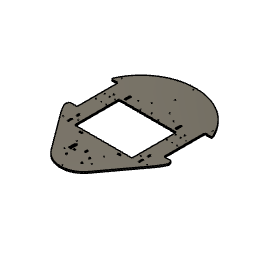
move_base_main_plate (Autodesk Fusion 360 design; units mm, degrees)
Autodesk Fusion 360 part; units mm, degrees
note: some values were not read from the file. Set by a fixed rule: which sketch regions a step uses.
sketch "スケッチ1" plane through (0, 0, 0) normal (0, 1, 0) x (1, 0, 0)
  circle A0 centre (0, 0) radius 210
  circle A1 centre (0, -210) radius 85
  line L0 (-168.7454, -125) -> (-68.3017, -260.5952)
  line L1 (68.3017, -260.5952) -> (168.7454, -125)
  circle A2 centre (0, 0) radius 200
  dimension "d1" = 420
  dimension "d2" = 210
  dimension "d3" = 170
  dimension "d4" = 400
  constraint coincident A0.centre A2.centre
  constraint vertical A0.centre A1.centre
  constraint tangent A0 L1
  constraint tangent A1 L1
  constraint tangent A1 L0
  constraint tangent A0 L0
  constraint coincident A0 L0.start
  constraint coincident A1 L0.end
  constraint coincident A1 L1.start
  constraint coincident A0 L1.end
  measures "d1" diameter of A0
  measures "d2" distance of A0.centre A1.centre
  measures "d3" diameter of A1
  measures "d4" diameter of A2
sketch "スケッチ2" plane through (0, 0, 0) normal (0, 1, 0) x (1, 0, 0)
  arc A0 (185.405, 75) -> (-185.405, 75) centre (0, 0) ccw
  arc A1 (-68.3017, -260.5952) -> (68.3017, -260.5952) centre (0, -210) ccw
  circle A2 centre (0, 0) radius 200
  line L0 (-185.405, 75) -> (-159, 75)
  line L1 (-159, 75) -> (-159, -75)
  line L2 (185.405, 75) -> (159, 75)
  line L3 (159, 75) -> (159, -75)
  line L4 (159, -75) -> (196.1505, -75)
  arc A3 (-196.1505, -75) -> (-168.7454, -125) centre (0, 0) ccw
  arc A4 (168.7454, -125) -> (196.1505, -75) centre (0, 0) ccw
  circle A5 centre (0, 0) radius 210
  line L5 (-168.7454, -125) -> (-68.3017, -260.5952)
  line L6 (68.3017, -260.5952) -> (168.7454, -125)
  line L7 (-196.1505, -75) -> (-159, -75)
  point P0 (-168.7454, -125)
  point P1 (-68.3017, -260.5952)
  point P2 (68.3017, -260.5952)
  point P3 (168.7454, -125)
  point P4 (0, -210)
  point P5 (-159, 0)
  point P6 (159, 0)
  dimension "d5" = 159
  dimension "d6" = 159
  dimension "d7" = 150
  dimension "d8" = 150
  constraint coincident A0.centre A2.centre
  constraint coincident A0.start A2
  constraint horizontal L0
  constraint perpendicular L0 L1
  constraint horizontal L2
  constraint perpendicular L2 L3
  constraint perpendicular L3 L4
  constraint coincident A3.start A5
  constraint coincident L4.end A5
  constraint coincident P0 A3.end
  constraint coincident P1 A1.start
  constraint coincident P2 A1.end
  constraint coincident P3 A4.start
  constraint horizontal L7
  constraint coincident L1.end L7.end
  constraint coincident L4.end A4.end
  constraint coincident A1.centre P4
  constraint midpoint L1 P5
  constraint midpoint L3 P6
  constraint horizontal P5 A0.centre
  constraint horizontal P6 A0.centre
  measures "d5" distance of L1 A0.centre
  measures "d6" distance of L3 A0.centre
  measures "d7" distance of L0.end L1.end
  measures "d8" distance of L2.end L3.end
extrude "押し出し1" add sketch "スケッチ2" along normal blind 5 contours A0 A2 L0 L1 L2 L3 L4 L7 | A2 L4 A3 A4 A5 L7 | A1 A5 L5 L6
sketch "スケッチ3" plane through (0, 5, 0) normal (0, 1, 0) x (-1, 0, 0)
  arc A0 (-185.405, -75) -> (185.405, -75) centre (0, 0) ccw
  line L0 (185.405, -75) -> (159, -75)
  line L1 (159, -75) -> (159, 75)
  line L2 (159, 75) -> (196.1505, 75)
  arc A1 (196.1505, 75) -> (168.7454, 125) centre (0, 0) ccw
  line L3 (168.7454, 125) -> (68.3017, 260.5952)
  arc A2 (68.3017, 260.5952) -> (-68.3017, 260.5952) centre (0, 210) ccw
  line L4 (-68.3017, 260.5952) -> (-168.7454, 125)
  arc A3 (-168.7454, 125) -> (-196.1505, 75) centre (0, 0) ccw
  line L5 (-196.1505, 75) -> (-159, 75)
  line L6 (-159, 75) -> (-159, -75)
  line L7 (-159, -75) -> (-185.405, -75)
  line L8 (-130, -70) -> (130, -70)
  line L9 (130, -70) -> (130, 150)
  line L10 (130, 150) -> (-130, 150)
  line L11 (-130, 150) -> (-130, -70)
  line L12 (-130, -70) -> (130, 150) construction
  line L13 (130, -70) -> (-130, 150) construction
  line L14 (149.05, -15.6) -> (110.95, -15.6)
  line L15 (110.95, -15.6) -> (110.95, 15.6)
  line L16 (110.95, 15.6) -> (149.05, 15.6)
  line L17 (149.05, 15.6) -> (149.05, -15.6)
  line L18 (-110.95, -15.6) -> (-149.05, -15.6)
  line L19 (-149.05, -15.6) -> (-149.05, 15.6)
  line L20 (-149.05, 15.6) -> (-110.95, 15.6)
  line L21 (-110.95, 15.6) -> (-110.95, -15.6)
  line L22 (0, 200) -> (0, 260)
  arc A4 (-166.2769, -96) -> (166.2769, -96) centre (0, 0) ccw
  line L23 (0, 0) -> (0, -192)
  line L24 (0, 0) -> (-166.2769, -96)
  line L25 (0, 0) -> (166.2769, -96)
  line L26 (0, 260) -> (0, 287)
  line L27 (154.1352, 131.2832) -> (61.8733, 255.8333)
  arc A5 (61.8733, 255.8333) -> (-61.8733, 255.8333) centre (0, 210) ccw
  line L28 (-154.1352, 131.2832) -> (-61.8733, 255.8333)
  line L29 (0, 210) -> (61.8733, 255.8333)
  line L30 (0, 210) -> (-61.8733, 255.8333)
  line L31 (-28, 216) -> (28, 216)
  line L32 (28, 216) -> (28, 244)
  line L33 (28, 244) -> (-28, 244)
  line L34 (-28, 244) -> (-28, 216)
  line L35 (-28, 216) -> (28, 244) construction
  line L36 (28, 216) -> (-28, 244) construction
  line L37 (114.5, 115) -> (114.5, -54.5)
  line L38 (114.5, -54.5) -> (-114.5, -54.5)
  line L39 (-114.5, -54.5) -> (-114.5, 115)
  line L40 (33, -73) -> (-33, -73)
  line L41 (-33, -73) -> (-33, -31.5)
  line L42 (-33, -31.5) -> (33, -31.5)
  line L43 (33, -31.5) -> (33, -73)
  line L44 (128, 122) -> (132, 122)
  line L45 (132, 122) -> (132, 138)
  line L46 (132, 138) -> (128, 138)
  line L47 (128, 138) -> (128, 122)
  line L48 (128, 122) -> (132, 138) construction
  line L49 (132, 122) -> (128, 138) construction
  line L50 (-132, 122) -> (-128, 122)
  line L51 (-128, 122) -> (-128, 138)
  line L52 (-128, 138) -> (-132, 138)
  line L53 (-132, 138) -> (-132, 122)
  line L54 (-132, 122) -> (-128, 138) construction
  line L55 (-128, 122) -> (-132, 138) construction
  point P0 (0, 40)
  point P1 (130, -15.6)
  point P2 (-130, -15.6)
  point P3 (110.95, 0)
  point P4 (-110.95, 0)
  point P5 (70, -70)
  point P6 (-70, -70)
  point P7 (130, -30)
  point P8 (130, 100)
  point P9 (70, 150)
  point P10 (-70, 150)
  point P11 (-130, 100)
  point P12 (-130, -30)
  point P13 (0, 230)
  point P14 (130, 15.6)
  point P15 (-130, 15.6)
  point P16 (65, -54.5)
  point P17 (-65, -54.5)
  point P18 (0, -40)
  point P19 (0, -73)
  point P20 (0, 256)
  point P21 (0, -125)
  point P22 (130, 130)
  point P23 (-130, 130)
  dimension "d13" = 260
  dimension "d14" = 220
  dimension "d15" = 40
  dimension "d16" = 70
  dimension "d17" = 60
  dimension "d18" = 70
  dimension "d19" = 70
  dimension "d20" = 50
  dimension "d21" = 60
  dimension "d22" = 38.1
  dimension "d23" = 31.2
  dimension "d24" = 192
  dimension "d25" = 60
  dimension "d26" = 60
  dimension "d28" = 27
  dimension "d29" = 77
  dimension "d30" = 155
  dimension "d31" = 155
  dimension "d32" = 53.5
  dimension "d33" = 230
  dimension "d34" = 28
  dimension "d35" = 56
  dimension "d56" = 15.5
  dimension "d57" = 15.5
  dimension "d58" = 15.5
  dimension "d59" = 115
  dimension "d60" = 65
  dimension "d61" = 65
  dimension "d65" = 66
  dimension "d66" = 41.5
  dimension "d99" = 85
  dimension "d100" = 40
  dimension "d116" = 4
  dimension "d117" = 16
  dimension "d134" = 3
  dimension "d145" = 130
  constraint horizontal L8
  constraint perpendicular L8 L9
  constraint parallel L8 L10
  constraint parallel L9 L11
  constraint coincident L12 P0
  constraint coincident L13 P0
  constraint vertical A0.centre P0
  constraint horizontal L14
  constraint vertical L15
  constraint horizontal L16
  constraint vertical L17
  constraint midpoint L14 P1
  constraint coincident L9 P1
  constraint horizontal L18
  constraint vertical L19
  constraint horizontal L20
  constraint vertical L21
  constraint midpoint L18 P2
  constraint coincident L11 P2
  constraint midpoint L21 P4
  constraint midpoint L15 P3
  constraint horizontal A0.centre P3
  constraint horizontal A0.centre P4
  constraint coincident L8 P5
  constraint coincident L8 P6
  constraint coincident L9 P8
  constraint coincident L10 P9
  constraint coincident L10 P10
  constraint coincident L11 P11
  constraint coincident L11 P12
  constraint vertical P5 P9
  constraint vertical P6 P10
  constraint horizontal P7 P12
  constraint horizontal P8 P11
  constraint parallel L9 L22
  constraint vertical A0.centre L22.start
  constraint equal L14 L18
  constraint equal L15 L19
  constraint coincident A0.centre A1.centre
  constraint coincident A4 L23.end
  constraint vertical L23
  constraint parallel L22 L26
  constraint coincident A2.centre A5.centre
  constraint coincident L27.end A5.start
  constraint coincident A5.end L28.end
  constraint tangent L27 A5
  constraint tangent A5 L28
  constraint parallel L4 L28
  constraint parallel L3 L27
  constraint horizontal L31
  constraint perpendicular L31 L32
  constraint parallel L31 L33
  constraint parallel L32 L34
  constraint coincident L35 P13
  constraint coincident L36 P13
  constraint vertical A0.centre P13
  constraint midpoint L16 P14
  constraint midpoint L20 P15
  constraint vertical L37
  constraint perpendicular L23 L38
  constraint perpendicular L38 L39
  constraint coincident L38 P16
  constraint coincident L38 P17
  constraint vertical A0.centre P18
  constraint horizontal L40
  constraint vertical L41
  constraint horizontal L42
  constraint vertical L43
  constraint coincident L40 P19
  constraint midpoint L40 P19
  constraint vertical A0.centre P19
  constraint coincident L26 P20
  constraint coincident L23 P21
  constraint horizontal L44
  constraint perpendicular L44 L45
  constraint parallel L44 L46
  constraint parallel L45 L47
  constraint coincident L48 P22
  constraint coincident L49 P22
  constraint coincident L9 P22
  constraint horizontal L50
  constraint perpendicular L50 L51
  constraint parallel L50 L52
  constraint parallel L51 L53
  constraint coincident L54 P23
  constraint coincident L55 P23
  constraint coincident L11 P23
  constraint equal L44 L50
  constraint equal L47 L51
  constraint horizontal L37.start L39.end
  constraint horizontal P22 P23
  measures "d13" distance of L8.start L8.end
  measures "d14" distance of L8.start L10.end
  measures "d15" distance of A0.centre P0
  measures "d16" vertical distance of P0 P7
  measures "d17" vertical distance of P0 P8
  measures "d18" horizontal distance of P0 P9
  measures "d19" horizontal distance of P0 P10
  measures "d20" distance of L10 L22.start
  measures "d21" distance of L22.start L22.end
  measures "d22" distance of L14.start L14.end
  measures "d23" distance of L14.end L15.end
  measures "d24" radius of A4
  measures "d25" angle of L23 L24
  measures "d26" angle of L23 L25
  measures "d28" distance of L22.end L26.end
  measures "d29" radius of A5
  measures "d30" distance of L28.start A5.end
  measures "d31" distance of L27.start L27.end
  measures "d33" distance of A0.centre P13
  measures "d34" distance of L31.start L33.end
  measures "d35" distance of L32.end L33.end
  measures "d56" distance of L9 L37
  measures "d57" distance of L11 L39
  measures "d58" distance of L8 L38
  measures "d59" vertical distance of A0.centre L37.start
  measures "d60" horizontal distance of A0.centre P16
  measures "d61" horizontal distance of A0.centre P17
  measures "d65" distance of L40.start L40.end
  measures "d66" distance of L40.start L42.end
  measures "d99" distance of P18 P21
  measures "d100" distance of A0.centre P18
  measures "d116" distance of L44.start L44.end
  measures "d117" distance of L44.end L45.end
  measures "d134" distance of L8 L40
  measures "d145" vertical distance of A0.centre P22
hole "穴1" at (-166.2769, 5, -96) at (0, 5, -192) at (166.2769, 5, -96) at (149.05, 5, -15.6) at (149.05, 5, 15.6) at (110.95, 5, -15.6) at (110.95, 5, 15.6) at (-110.95, 5, -15.6) at (-149.05, 5, -15.6) at (-149.05, 5, 15.6) at (-110.95, 5, 15.6) at (-130, 5, -15.6) at (130, 5, -15.6) at (130, 5, 15.6) at (-130, 5, 15.6) at (-154.1352, 5, 131.2832) at (0, 5, 287) at (154.1352, 5, 131.2832) at (-114.5, 5, 115) at (-65, 5, -54.5) at (65, 5, -54.5) at (114.5, 5, 115) at (-33, 5, -31.5) at (33, 5, -31.5) at (33, 5, -73) at (-33, 5, -73) at (0, 5, -40) at (0, 5, -125) direction (0, -1, 0) diameter 3.2 end through all
sketch "スケッチ4" plane through (0, 5, 0) normal (0, 1, 0) x (-1, 0, 0)
  circle A0 centre (0, 287) radius 1.6
  circle A1 centre (130, 15.6) radius 1.6
  circle A2 centre (-130, -15.6) radius 1.6
  circle A3 centre (110.95, 15.6) radius 1.6
  circle A4 centre (149.05, -15.6) radius 1.6
  circle A5 centre (-110.95, 15.6) radius 1.6
  circle A6 centre (-149.05, 15.6) radius 1.6
  circle A7 centre (-166.2769, -96) radius 1.6
  circle A8 centre (166.2769, -96) radius 1.6
  circle A9 centre (0, -192) radius 1.6
  circle A10 centre (-149.05, -15.6) radius 1.6
  circle A11 centre (-110.95, -15.6) radius 1.6
  circle A12 centre (110.95, -15.6) radius 1.6
  circle A13 centre (149.05, 15.6) radius 1.6
  circle A14 centre (130, -15.6) radius 1.6
  circle A15 centre (-130, 15.6) radius 1.6
  circle A16 centre (154.1352, 131.2832) radius 1.6
  circle A17 centre (-154.1352, 131.2832) radius 1.6
  arc A18 (-185.405, -75) -> (185.405, -75) centre (0, 0) ccw
  line L0 (185.405, -75) -> (159, -75)
  line L1 (159, -75) -> (159, 75)
  line L2 (159, 75) -> (196.1505, 75)
  arc A19 (196.1505, 75) -> (168.7454, 125) centre (0, 0) ccw
  line L3 (168.7454, 125) -> (68.3017, 260.5952)
  arc A20 (68.3017, 260.5952) -> (-68.3017, 260.5952) centre (0, 210) ccw
  line L4 (-68.3017, 260.5952) -> (-168.7454, 125)
  arc A21 (-168.7454, 125) -> (-196.1505, 75) centre (0, 0) ccw
  line L5 (-196.1505, 75) -> (-159, 75)
  line L6 (-159, 75) -> (-159, -75)
  line L7 (-159, -75) -> (-185.405, -75)
  line L8 (127.85, -34) -> (132.15, -34)
  line L9 (132.15, -34) -> (132.15, -26)
  line L10 (132.15, -26) -> (127.85, -26)
  line L11 (127.85, -26) -> (127.85, -34)
  line L12 (127.85, -34) -> (132.15, -26) construction
  line L13 (132.15, -34) -> (127.85, -26) construction
  circle A22 centre (130, -34) radius 2.15
  circle A23 centre (130, -26) radius 2.15
  line L14 (127.85, 96) -> (132.15, 96)
  line L15 (132.15, 96) -> (132.15, 104)
  line L16 (132.15, 104) -> (127.85, 104)
  line L17 (127.85, 104) -> (127.85, 96)
  line L18 (127.85, 96) -> (132.15, 104) construction
  line L19 (132.15, 96) -> (127.85, 104) construction
  line L20 (-132.15, 96) -> (-127.85, 96)
  line L21 (-127.85, 96) -> (-127.85, 104)
  line L22 (-127.85, 104) -> (-132.15, 104)
  line L23 (-132.15, 104) -> (-132.15, 96)
  line L24 (-132.15, 96) -> (-127.85, 104) construction
  line L25 (-127.85, 96) -> (-132.15, 104) construction
  line L26 (-132.15, -34) -> (-127.85, -34)
  line L27 (-127.85, -34) -> (-127.85, -26)
  line L28 (-127.85, -26) -> (-132.15, -26)
  line L29 (-132.15, -26) -> (-132.15, -34)
  line L30 (-132.15, -34) -> (-127.85, -26) construction
  line L31 (-127.85, -34) -> (-132.15, -26) construction
  line L32 (66, 147.85) -> (74, 147.85)
  line L33 (74, 147.85) -> (74, 152.15)
  line L34 (74, 152.15) -> (66, 152.15)
  line L35 (66, 152.15) -> (66, 147.85)
  line L36 (66, 147.85) -> (74, 152.15) construction
  line L37 (74, 147.85) -> (66, 152.15) construction
  line L38 (-74, 147.85) -> (-66, 147.85)
  line L39 (-66, 147.85) -> (-66, 152.15)
  line L40 (-66, 152.15) -> (-74, 152.15)
  line L41 (-74, 152.15) -> (-74, 147.85)
  line L42 (-74, 147.85) -> (-66, 152.15) construction
  line L43 (-66, 147.85) -> (-74, 152.15) construction
  circle A24 centre (-130, -34) radius 2.15
  circle A25 centre (-130, -26) radius 2.15
  circle A26 centre (-130, 96) radius 2.15
  circle A27 centre (-130, 104) radius 2.15
  circle A28 centre (-74, 150) radius 2.15
  circle A29 centre (-66, 150) radius 2.15
  circle A30 centre (66, 150) radius 2.15
  circle A31 centre (74, 150) radius 2.15
  circle A32 centre (130, 96) radius 2.15
  circle A33 centre (130, 104) radius 2.15
  line L44 (-2.15, 196) -> (2.15, 196)
  line L45 (2.15, 196) -> (2.15, 204)
  line L46 (2.15, 204) -> (-2.15, 204)
  line L47 (-2.15, 204) -> (-2.15, 196)
  line L48 (-2.15, 196) -> (2.15, 204) construction
  line L49 (2.15, 196) -> (-2.15, 204) construction
  circle A34 centre (0, 196) radius 2.15
  circle A35 centre (0, 204) radius 2.15
  circle A36 centre (-65, -54.5) radius 1.6
  circle A37 centre (114.5, 115) radius 1.6
  circle A38 centre (65, -54.5) radius 1.6
  circle A39 centre (-114.5, 115) radius 1.6
  circle A40 centre (-33, -73) radius 1.6
  circle A41 centre (33, -31.5) radius 1.6
  circle A42 centre (-33, -31.5) radius 1.6
  circle A43 centre (33, -73) radius 1.6
  circle A44 centre (0, -40) radius 1.6
  circle A45 centre (0, -125) radius 1.6
  point P0 (130, -30)
  point P1 (130, -30)
  point P2 (130, 100)
  point P3 (-130, 100)
  point P4 (-130, -30)
  point P5 (70, 150)
  point P6 (-70, 150)
  point P7 (130, 100)
  point P8 (70, 150)
  point P9 (-70, 150)
  point P10 (-130, 100)
  point P11 (-130, -30)
  point P12 (0, 200)
  point P13 (0, 200)
  dimension "d39" = 4.3
  dimension "d40" = 8
  constraint horizontal L8
  constraint perpendicular L8 L9
  constraint parallel L8 L10
  constraint parallel L9 L11
  constraint coincident L12 P1
  constraint coincident L13 P1
  constraint coincident P1 P0
  constraint midpoint L8 A22.centre
  constraint coincident L8.start A22
  constraint midpoint L10 A23.centre
  constraint coincident L10.end A23
  constraint horizontal L14
  constraint perpendicular L14 L15
  constraint parallel L14 L16
  constraint parallel L15 L17
  constraint coincident L18 P7
  constraint coincident L19 P7
  constraint horizontal L20
  constraint perpendicular L20 L21
  constraint parallel L20 L22
  constraint parallel L21 L23
  constraint coincident L24 P10
  constraint coincident L25 P10
  constraint horizontal L26
  constraint perpendicular L26 L27
  constraint parallel L26 L28
  constraint parallel L27 L29
  constraint coincident L30 P11
  constraint coincident L31 P11
  constraint horizontal L32
  constraint perpendicular L32 L33
  constraint parallel L32 L34
  constraint parallel L33 L35
  constraint coincident L36 P8
  constraint coincident L37 P8
  constraint horizontal L38
  constraint perpendicular L38 L39
  constraint parallel L38 L40
  constraint parallel L39 L41
  constraint coincident L42 P9
  constraint coincident L43 P9
  constraint coincident P7 P2
  constraint coincident P8 P5
  constraint coincident P9 P6
  constraint coincident P10 P3
  constraint coincident P11 P4
  constraint equal L11 L17
  constraint equal L17 L32
  constraint equal L32 L38
  constraint equal L21 L27
  constraint equal L20 L28
  constraint equal L35 L39
  constraint equal L10 L14
  constraint equal L16 L33
  constraint midpoint L26 A24.centre
  constraint coincident L26.start A24
  constraint midpoint L28 A25.centre
  constraint coincident L28.end A25
  constraint midpoint L20 A26.centre
  constraint coincident L20.start A26
  constraint midpoint L22 A27.centre
  constraint coincident L22.end A27
  constraint midpoint L41 A28.centre
  constraint coincident L38.start A28
  constraint midpoint L39 A29.centre
  constraint coincident L38.end A29
  constraint midpoint L35 A30.centre
  constraint coincident L32.start A30
  constraint midpoint L33 A31.centre
  constraint coincident L32.end A31
  constraint midpoint L14 A32.centre
  constraint coincident L14.start A32
  constraint midpoint L16 A33.centre
  constraint coincident L16.end A33
  constraint horizontal L44
  constraint perpendicular L44 L45
  constraint parallel L44 L46
  constraint parallel L45 L47
  constraint coincident L48 P13
  constraint coincident L49 P13
  constraint coincident P13 P12
  constraint equal L35 L44
  constraint equal L32 L45
  constraint midpoint L44 A34.centre
  constraint coincident L44.start A34
  constraint midpoint L46 A35.centre
  constraint coincident L46.end A35
  measures "d39" distance of L8.start L8.end
  measures "d40" distance of L8.start L10.end
extrude "押し出し2" cut sketch "スケッチ4" against normal through all contours L14 A32 | L15 L17 A32 A33 | L14 A32 | L16 A33 | L16 A33 | L20 A26 | L21 L23 A26 A27 | L20 A26 | L22 A27 | L22 A27 | L32 L34 A30 A31 | L35 A30 | L35 A30 | L33 A31 | L33 A31 | L38 L40 A28 A29 | L41 A28 | L41 A28 | L39 A29 | L39 A29 | L44 A34 | L45 L47 A34 A35 | L44 A34 | L46 A35 | L46 A35
hole "穴2" at (-28, 5, 244) at (28, 5, 244) at (28, 5, 216) at (-28, 5, 216) direction (0, -1, 0) diameter 6.3 end through all
sketch "スケッチ5" plane through (0, 5, 0) normal (0, 1, 0) x (-1, 0, 0)
  circle A0 centre (-28, 216) radius 3.15
  circle A1 centre (28, 244) radius 3.15
  circle A2 centre (-28, 244) radius 3.15
  circle A3 centre (28, 216) radius 3.15
  line L0 (74, 147.85) -> (66, 147.85)
  arc A4 (66, 152.15) -> (66, 147.85) centre (66, 150) ccw
  line L1 (66, 152.15) -> (74, 152.15)
  arc A5 (74, 147.85) -> (74, 152.15) centre (74, 150) ccw
  line L2 (132.15, 104) -> (132.15, 96)
  arc A6 (127.85, 96) -> (132.15, 96) centre (130, 96) ccw
  line L3 (127.85, 96) -> (127.85, 104)
  arc A7 (132.15, 104) -> (127.85, 104) centre (130, 104) ccw
  line L4 (-66, 147.85) -> (-74, 147.85)
  arc A8 (-74, 152.15) -> (-74, 147.85) centre (-74, 150) ccw
  line L5 (-74, 152.15) -> (-66, 152.15)
  arc A9 (-66, 147.85) -> (-66, 152.15) centre (-66, 150) ccw
  line L6 (-127.85, 103.9983) -> (-127.85, 96)
  arc A10 (-132.15, 96) -> (-127.85, 96) centre (-130, 96) ccw
  line L7 (-132.15, 96) -> (-132.15, 104)
  arc A11 (-127.85, 103.9983) -> (-132.15, 104) centre (-130, 104) ccw
  line L8 (2.15, 204) -> (2.15, 196)
  arc A12 (-2.15, 196) -> (2.15, 196) centre (0, 196) ccw
  line L9 (-2.15, 196) -> (-2.15, 204)
  arc A13 (2.15, 204) -> (-2.15, 204) centre (0, 204) ccw
  circle A14 centre (0, 287) radius 1.6
  circle A15 centre (130, 15.6) radius 1.6
  circle A16 centre (-130, -15.6) radius 1.6
  circle A17 centre (110.95, 15.6) radius 1.6
  circle A18 centre (149.05, -15.6) radius 1.6
  circle A19 centre (-110.95, 15.6) radius 1.6
  circle A20 centre (-149.05, 15.6) radius 1.6
  circle A21 centre (-166.2769, -96) radius 1.6
  circle A22 centre (166.2769, -96) radius 1.6
  circle A23 centre (0, -192) radius 1.6
  circle A24 centre (-149.05, -15.6) radius 1.6
  circle A25 centre (-110.95, -15.6) radius 1.6
  circle A26 centre (110.95, -15.6) radius 1.6
  circle A27 centre (149.05, 15.6) radius 1.6
  circle A28 centre (130, -15.6) radius 1.6
  circle A29 centre (-130, 15.6) radius 1.6
  circle A30 centre (154.1352, 131.2832) radius 1.6
  circle A31 centre (-154.1352, 131.2832) radius 1.6
  arc A32 (-185.405, -75) -> (185.405, -75) centre (0, 0) ccw
  line L10 (185.405, -75) -> (159, -75)
  line L11 (159, -75) -> (159, 75)
  line L12 (159, 75) -> (196.1505, 75)
  arc A33 (196.1505, 75) -> (168.7454, 125) centre (0, 0) ccw
  line L13 (168.7454, 125) -> (68.3017, 260.5952)
  arc A34 (68.3017, 260.5952) -> (-68.3017, 260.5952) centre (0, 210) ccw
  line L14 (-68.3017, 260.5952) -> (-168.7454, 125)
  arc A35 (-168.7454, 125) -> (-196.1505, 75) centre (0, 0) ccw
  line L15 (-196.1505, 75) -> (-159, 75)
  line L16 (-159, 75) -> (-159, -75)
  line L17 (-159, -75) -> (-185.405, -75)
  line L18 (-105, -25) -> (-105, 138)
  line L19 (-105, 138) -> (105, 138)
  line L20 (105, 138) -> (105, -25)
  circle A36 centre (-65, -54.5) radius 1.6
  circle A37 centre (114.5, 115) radius 1.6
  circle A38 centre (65, -54.5) radius 1.6
  circle A39 centre (-114.5, 115) radius 1.6
  circle A40 centre (-33, -73) radius 1.6
  circle A41 centre (33, -31.5) radius 1.6
  circle A42 centre (-33, -31.5) radius 1.6
  circle A43 centre (33, -73) radius 1.6
  line L21 (96, -35) -> (90, -35)
  line L22 (90, -35) -> (90, -55)
  line L23 (90, -55) -> (96, -55)
  line L24 (96, -55) -> (96, -35)
  line L25 (-90, -35) -> (-96, -35)
  line L26 (-96, -35) -> (-96, -55)
  line L27 (-96, -55) -> (-90, -55)
  line L28 (-90, -55) -> (-90, -35)
  circle A44 centre (0, -40) radius 1.6
  circle A45 centre (0, -125) radius 1.6
  line L29 (105, -25) -> (-105, -25)
  line L30 (50, 185) -> (-50, 185)
  line L31 (-50, 185) -> (-50, 230)
  line L32 (-50, 230) -> (50, 230)
  line L33 (50, 230) -> (50, 185)
  line L34 (45, 195) -> (37, 195)
  line L35 (37, 195) -> (37, 220)
  line L36 (37, 220) -> (45, 220)
  line L37 (45, 220) -> (45, 195)
  point P0 (0, -7)
  point P1 (0, 185)
  dimension "d45" = 138
  dimension "d49" = 105
  dimension "d50" = 105
  dimension "d76" = 35
  dimension "d77" = 20
  dimension "d78" = 6
  dimension "d79" = 90
  dimension "d80" = 90
  dimension "d114" = 25
  dimension "d135" = 100
  dimension "d136" = 45
  dimension "d137" = 185
  dimension "d141" = 8
  dimension "d142" = 5
  dimension "d143" = 10
  dimension "d144" = 10
  constraint perpendicular L18 L19
  constraint perpendicular L19 L20
  constraint horizontal L21
  constraint vertical L22
  constraint horizontal L23
  constraint vertical L24
  constraint horizontal L25
  constraint vertical L26
  constraint horizontal L27
  constraint vertical L28
  constraint collinear L21 L25
  constraint equal L22 L26
  constraint equal L23 L27
  constraint vertical L18
  constraint perpendicular L20 L29
  constraint vertical A32.centre P0
  constraint coincident L18.start L29.end
  constraint horizontal L30
  constraint vertical L31
  constraint horizontal L32
  constraint vertical L33
  constraint midpoint L30 P1
  constraint vertical A32.centre P1
  constraint horizontal L34
  constraint vertical L35
  constraint horizontal L36
  constraint vertical L37
  measures "d45" distance of L19 A32.centre
  measures "d49" distance of L20 A32.centre
  measures "d50" distance of L18 A32.centre
  measures "d76" distance of A32.centre L25
  measures "d77" distance of L25.end L26.end
  measures "d78" distance of L26.end L27.end
  measures "d79" distance of A32.centre L28
  measures "d80" distance of A32.centre L22
  measures "d114" distance of A32.centre L29
  measures "d135" distance of L30.start L30.end
  measures "d136" distance of L30.end L31.end
  measures "d137" distance of A32.centre P1
  measures "d141" distance of L34.start L34.end
  measures "d142" distance of L33 L37
  measures "d143" distance of L30 L34
  measures "d144" distance of L32 L36
extrude "押し出し3" cut sketch "スケッチ5" against normal through all contours L18 L19 L20 L29 | L21 L22 L23 L24 | L25 L26 L27 L28 | L34 L35 L36 L37
hole "穴3" at (-130, 5, -30) at (130, 5, -30) direction (0, -1, 0) diameter 4.2 end through all
chamfer "面取り1" distance 15 distance2 10 1 edges at (196.1505, 2.5, 75) measured on face at (172.4502, 1.6667, 119.837)
chamfer "面取り2" distance 10 distance2 15 1 edges at (-196.1505, 2.5, 75) measured on face at (-183.767, 1.6667, 75)
fillet "フィレット2" radius 3 14 edges at (-185.405, 2.5, -75) (185.405, 2.5, -75) (105, 2.5, 138) (-105, 2.5, 138) (190.2963, 2.5, 88.8105) (186.1505, 2.5, 75) (-186.1505, 2.5, 75) (-190.2963, 2.5, 88.8105) (-105, 2.5, -25) (159, 2.5, 75) (159, 2.5, -75) (-159, 2.5, 75) (-159, 2.5, -75) (105, 2.5, -25)
extrude "押し出し4" cut sketch "スケッチ3" against normal through all contours L11 L50 L52 L53 | L11 L50 L51 L52 | L9 L44 L45 L46 | L9 L44 L46 L47
hole "穴5" at (-50, 5, 185) at (-50, 5, 230) at (50, 5, 230) at (50, 5, 185) direction (0, -1, 0) diameter 3.2 end through all
